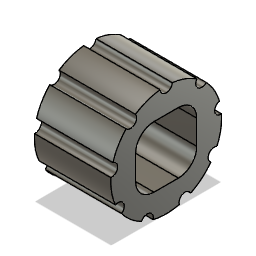
Mud Guard Clamp v1 (Autodesk Fusion 360 design; units mm, degrees)
Autodesk Fusion 360 part; units mm, degrees
sketch "Sketch1" plane through (0, 0, 0) normal (1, 0, 0) x (0, 0, -1)
  line L0 (-10, 10) -> (10, 10)
  line L1 (10, 10) -> (10, -10)
  line L2 (10, -10) -> (-10, -10)
  line L3 (-10, -10) -> (-10, 10)
  line L4 (-10, 10) -> (10, -10) construction
  line L5 (10, 10) -> (-10, -10) construction
  circle A0 centre (0, 0) radius 14.1421 construction
  circle A1 centre (0, 0) radius 18.1421
  circle A2 centre (0, 18.1421) radius 2
  circle A3 centre (-11.6615, 13.8977) radius 2
  circle A4 centre (-17.8665, 3.1503) radius 2
  circle A5 centre (-15.7116, -9.0711) radius 2
  circle A6 centre (-6.205, -17.048) radius 2
  circle A7 centre (6.205, -17.048) radius 2
  circle A8 centre (15.7116, -9.0711) radius 2
  circle A9 centre (17.8665, 3.1503) radius 2
  circle A10 centre (11.6615, 13.8977) radius 2
  circle A11 centre (0, 0) radius 20.1421 construction
  circle A12 centre (0, 0) radius 24.1421
  dimension "d1" = 20
  dimension "d2" = 20
  dimension "d3" = 4
  dimension "d4" = 4
  dimension "d6" = 360
  dimension "d7" = 4
  constraint horizontal L0
  constraint perpendicular L0 L1
  constraint parallel L0 L2
  constraint parallel L1 L3
  constraint coincident L4 A0.centre
  constraint coincident L5 A0.centre
  constraint coincident A0.centre A1.centre
  constraint coincident L0.end A0
  constraint coincident A1 A2.centre
  constraint vertical A0.centre A2.centre
  constraint tangent A10 A11
  measures "d1" distance of L1.end L2.end
  measures "d2" distance of L0.end L1.end
  measures "d4" diameter of A2
extrude "Extrude1" add sketch "Sketch1" along normal blind 25 contours A1 A2 A3 A4 A5 A6 A7 A8 A9 A10
fillet "Fillet1" radius 6 4 edges at (12.5, 10, 10) (12.5, -10, 10) (12.5, -10, -10) (12.5, 10, -10)
sketch "Sketch4" plane through (-160, 0, 0) normal (-1, 0, 0) x (0, 0, 1)
  line L0 (-4, 17) -> (15, 5)
  line L1 (15, 5) -> (14, -7)
  line L2 (14, -7) -> (1, -17)
  line L3 (1, -17) -> (-12, -12)
  line L4 (-12, -12) -> (-14.488, 8.6817)
  line L5 (-14.488, 8.6817) -> (-4, 17)
sketch "Sketch5" plane through (-160, 0, 0) normal (-1, 0, 0) x (0, 0, 1)
  arc A0 (-14.6176, -10.7454) -> (-8.0438, -16.2614) centre (0, 0) ccw
  arc A1 (-4.2907, -17.6274) -> (-8.0438, -16.2614) centre (-6.205, -17.048) ccw
  arc A2 (-4.2907, -17.6274) -> (4.2907, -17.6274) centre (0, 0) ccw
  arc A3 (8.0438, -16.2614) -> (4.2907, -17.6274) centre (6.205, -17.048) ccw
  arc A4 (8.0438, -16.2614) -> (14.6176, -10.7454) centre (0, 0) ccw
  arc A5 (16.6146, -7.2865) -> (14.6176, -10.7454) centre (15.7116, -9.0711) ccw
  arc A6 (16.6146, -7.2865) -> (18.1047, 1.1646) centre (0, 0) ccw
  arc A7 (17.4112, 5.0978) -> (18.1047, 1.1646) centre (17.8665, 3.1503) ccw
  arc A8 (17.4112, 5.0978) -> (13.1204, 12.5296) centre (0, 0) ccw
  arc A9 (10.0609, 15.0969) -> (13.1204, 12.5296) centre (11.6615, 13.8977) ccw
  arc A10 (10.0609, 15.0969) -> (1.997, 18.0319) centre (0, 0) ccw
  arc A11 (-1.997, 18.0319) -> (1.997, 18.0319) centre (0, 18.1421) ccw
  arc A12 (-1.997, 18.0319) -> (-10.0609, 15.0969) centre (0, 0) ccw
  arc A13 (-13.1204, 12.5296) -> (-10.0609, 15.0969) centre (-11.6615, 13.8977) ccw
  arc A14 (-13.1204, 12.5296) -> (-17.4112, 5.0978) centre (0, 0) ccw
  arc A15 (-18.1047, 1.1646) -> (-17.4112, 5.0978) centre (-17.8665, 3.1503) ccw
  arc A16 (-18.1047, 1.1646) -> (-16.6146, -7.2865) centre (0, 0) ccw
  arc A17 (-14.6176, -10.7454) -> (-16.6146, -7.2865) centre (-15.7116, -9.0711) ccw
  line L0 (-6.3241, 11) -> (6.3241, 11)
  line L1 (11, 6.3241) -> (11, -6.3241)
  line L2 (6.3241, -11) -> (-6.3241, -11)
  line L3 (-11, -6.3241) -> (-11, 6.3241)
  line L4 (-11, 11) -> (11, -11) construction
  line L5 (11, 11) -> (-11, -11) construction
  line L6 (11, -6.3241) -> (6.3241, -11)
  line L7 (-6.3241, -11) -> (-11, -6.3241)
  line L8 (-17.3241, 0) -> (17.3241, 0) construction
  line L9 (0, 17.3241) -> (0, -17.3241) construction
  line L10 (6.3241, 11) -> (11, 6.3241)
  line L11 (-11, 6.3241) -> (-6.3241, 11)
  dimension "d96" = 22
  dimension "d97" = 22
  dimension "d98" = 24.5
  dimension "d99" = 24.5
  constraint horizontal L0
  constraint perpendicular L0 L1
  constraint parallel L0 L2
  constraint parallel L1 L3
  constraint coincident L4 A0.centre
  constraint coincident L5 A0.centre
  constraint coincident A0.centre A2.centre
  constraint parallel L6 L11
  constraint coincident L8 A0.centre
  constraint coincident L9 A0.centre
  measures "d96" distance of L4.end L5.end
  measures "d97" distance of L5.start L4.end
  measures "d98" distance of L8.end L9.end
  measures "d99" distance of L9.start L8.end
sketch "Sketch6" plane through (0, 0, 0) normal (0, 0, 1) x (1, 0, 0)
sketch "Sketch8" plane through (0, 0, 0) normal (-1, 0, 0) x (0, 0, 1)
  arc A0 (23.743, -4.3718) -> (6.1466, 23.3466) centre (0, 0) ccw
  arc A1 (6.1466, 23.3466) -> (-24.0592, -1.9991) centre (0, 0) ccw
  arc A2 (-24.0592, -1.9991) -> (0.1825, -24.1414) centre (0, 0) ccw
  arc A3 (0.1825, -24.1414) -> (23.743, -4.3718) centre (0, 0) ccw
  arc A4 (16.6857, -7.6172) -> (18.2847, 1.451) centre (0, 0) ccw
  arc A5 (16.6857, -7.6172) -> (14.9396, -10.6416) centre (15.7116, -9.0711) ccw
  arc A6 (7.8857, -16.5605) -> (14.9396, -10.6416) centre (0, 0) ccw
  arc A7 (7.8857, -16.5605) -> (4.6041, -17.7549) centre (6.205, -17.048) ccw
  arc A8 (-4.6041, -17.7549) -> (4.6041, -17.7549) centre (0, 0) ccw
  arc A9 (-4.6041, -17.7549) -> (-7.8857, -16.5605) centre (-6.205, -17.048) ccw
  arc A10 (-14.9396, -10.6416) -> (-7.8857, -16.5605) centre (0, 0) ccw
  arc A11 (-14.9396, -10.6416) -> (-16.6857, -7.6172) centre (-15.7116, -9.0711) ccw
  arc A12 (-18.2847, 1.451) -> (-16.6857, -7.6172) centre (0, 0) ccw
  arc A13 (-18.2847, 1.451) -> (-17.6782, 4.8902) centre (-17.8665, 3.1503) ccw
  arc A14 (-13.0741, 12.8647) -> (-17.6782, 4.8902) centre (0, 0) ccw
  arc A15 (-13.0741, 12.8647) -> (-10.399, 15.1095) centre (-11.6615, 13.8977) ccw
  arc A16 (-1.7461, 18.2588) -> (-10.399, 15.1095) centre (0, 0) ccw
  arc A17 (-1.7461, 18.2588) -> (1.7461, 18.2588) centre (0, 18.1421) ccw
  arc A18 (10.399, 15.1095) -> (1.7461, 18.2588) centre (0, 0) ccw
  arc A19 (10.399, 15.1095) -> (13.0741, 12.8647) centre (11.6615, 13.8977) ccw
  arc A20 (17.6782, 4.8902) -> (13.0741, 12.8647) centre (0, 0) ccw
  arc A21 (17.6782, 4.8902) -> (18.2847, 1.451) centre (17.8665, 3.1503) ccw
equation "Diameter = 220 mm"
equation "Width = 75 mm"
equation "Thickness_experimental = 5 mm"
equation "Front_Bias = 25 deg"
equation "Rear_Bias = 15 deg"
equation "Roundness = 0.5" comment "Value between 0 and 1"
equation "Corner_Radius = 20 mm"
